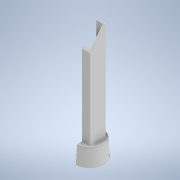
# Autodesk Inventor part: nozzle
Saved by Autodesk Inventor 2020.2 (Build 242310000, 310)
## iProperties
Created: 2020-09-23
Part Number: nozzle
Material: Generic
Document SubType Name: Modeling
Designer: Amaan Khalid
Density: 1 g/cm^3
Appearance: Default
Author: Amaan Khalid
Autodesk Inventor part; units mm, degrees
sketch "Sketch1" plane through (0, 0, 0) normal (1, 0, 0) x (0, 1, 0)
  line L0 (1.2879, 8.5778) -> (-61.8197, 8.5778)
  line L1 (-61.8197, 8.5778) -> (-61.8197, -4.1222)
  line L2 (-61.8197, -4.1222) -> (1.6803, -4.1222)
  line L3 (1.6803, -4.1222) -> (7.0029, -4.1222)
  line L4 (1.2879, 8.5778) -> (1.4492, 8.5778)
  line L5 (7.0029, -4.1222) -> (15.0709, -4.1222)
  line L6 (15.4791, -3.0007) -> (1.8574, 8.4293)
  arc A0 (1.8574, 8.4293) -> (1.4492, 8.5778) centre (1.4492, 7.9428) ccw
  arc A1 (15.0709, -4.1222) -> (15.4791, -3.0007) centre (15.0709, -3.4872) ccw
  point P0 (0, 0)
  point P1 (1.6803, 8.5778)
  point P2 (8.0303, -4.1222)
  dimension "d0" = 63.5
  dimension "d1" = 12.7
  dimension "d2" = 63.5
  dimension "d3" = 6.35
  dimension "d17" = 0.635
  constraints: 14 end point, 4 horizontal, 4 point on circle, 4 point on line, 4 tangent, 2 centre point, 1 equal radius, 1 perpendicular, 1 vertical
  measures "d0" distance of point (1.68, 8.578) L0.end
  measures "d1" distance of L0.end L1.end
  measures "d2" distance of L1.end L2.end
  measures "d3" distance of L2.end point (8.03, -4.122)
  measures "d17" radius of A0
extrude "Extrusion1" add sketch "Sketch1" along normal blind 12.7
sketch "Sketch2" plane through (0, -61.8197, -4.1222) normal (0, -1, 0) x (1, 0, 0)
  line L0 (12.7, 12.349) -> (12.7, 12.7) projected
  line L1 (0, 12.7) -> (0, 0) projected
  line L2 (12.7, 12.7) -> (0, 12.7)
  line L3 (0, 12.7) -> (0, 0)
  line L4 (0, 0) -> (12.7, 0)
  line L5 (12.7, 0) -> (12.7, 12.7)
  line L6 (11.43, 11.43) -> (1.27, 11.43)
  line L7 (1.27, 11.43) -> (1.27, 1.27)
  line L8 (1.27, 1.27) -> (11.43, 1.27)
  line L9 (11.43, 1.27) -> (11.43, 11.43)
  point P0 (0, 4.1222)
  dimension "d7" = 1.27
  constraints: 16 end point, 4 parallel, 2 perpendicular, 1 horizontal, 3 other
  measures "d7" distance between parallel lines of L5 L9
extrude "Extrusion2" cut sketch "Sketch2" against normal through all contours L9 L8 L7 L6
fillet "Fillet1" radius 0.635 14 edges at (12.7, -30.1852, 8.5778) (12.7, -61.8197, 2.2278) (12.7, -23.3744, -4.1222) (12.7, 15.6676, -3.7043) (12.7, 8.6682, 2.7143) (12.7, 1.6664, 8.5395) (0, -30.1852, 8.5778) (0, -61.8197, 2.2278) (0, -23.3744, -4.1222) (0, 15.6676, -3.7043) (0, 8.6682, 2.7143) (0, 1.6664, 8.5395) (6.35, -61.8197, 8.5778) (6.35, -61.8197, -4.1222)
ref_plane "Work Plane1" through (0, -63.5, 0) normal (0, 1, 0) x (-1, 0, 0)
sketch "Sketch6" plane through (0, -63.5, 0) normal (0, 1, 0) x (-1, 0, 0)
  circle A0 centre (-6.35, 2.2278) radius 10.0838
  line L0 (-11.43, 7.3078) -> (-1.27, 7.3078) projected
  line L1 (-1.27, 7.3078) -> (-11.43, 7.3078)
  line L2 (-11.43, -2.8522) -> (-11.43, 7.3078) projected
  line L3 (-11.43, 7.3078) -> (-11.43, -2.8522)
  line L4 (-11.43, -2.8522) -> (-1.27, -2.8522)
  line L5 (-1.27, 7.3078) -> (-1.27, -2.8522) projected
  line L6 (-1.27, -2.8522) -> (-1.27, 7.3078)
  point P0 (0, 0)
  point P1 (-1.905, 6.6728)
  point P2 (-1.905, -2.2172)
  point P3 (-10.795, 6.6728)
  point P4 (-10.795, -2.2172)
  point P5 (-1.27, -2.8522)
  constraints: 8 end point, 2 collinear, 1 centre point, 1 horizontal, 1 vertical
extrude "Extrusion4" add sketch "Sketch6" along normal up to surface (2.3153 mm away)
ref_plane "Work Plane2" through (0, 0, 2.2352) normal (0, 0, 1) x (1, 0, 0)
sketch "Sketch7" plane through (0, 0, 2.2352) normal (0, 0, 1) x (1, 0, 0)
  line L0 (-3.7338, -63.5) -> (-3.7338, -61.1847) projected
  line L1 (-3.7338, -63.5) -> (-3.7338, -71.12)
  line L2 (1.27, -63.5) -> (1.27, 3.1938) projected
  line L3 (-3.7338, -71.12) -> (1.27, -63.5)
  line L4 (0.635, -61.1847) -> (12.065, -61.1847) projected
  line L5 (6.35, -61.1847) -> (6.35, -66.8359)
  line L6 (-3.7338, -63.5) -> (1.27, -63.5)
  point P0 (0, 0)
  dimension "d21" = 7.62
  constraints: 8 end point, 1 collinear, 1 midpoint, 1 point on line, 1 vertical
  measures "d21" distance of L1.start L1.end
sketch "Sketch8" plane through (0, 0, 2.2352) normal (0, 0, 1) x (1, 0, 0)
  point P0 (0, 0)
sketch "Sketch9" plane through (0, 0, 2.2352) normal (0, 0, 1) x (1, 0, 0)
  point P0 (0, 0)
ref_plane "Work Plane3" through (0, 0, 0) normal (1, 0, 0) x (0, 1, 0)
sketch "Sketch10" plane through (0, 0, 0) normal (1, 0, 0) x (0, 1, 0)
  point P0 (0, 0)
ref_plane "Work Plane4" through (6.35, 0, 0) normal (1, 0, 0) x (0, 1, 0)
sketch "Sketch11" plane through (0, 0, 0) normal (1, 0, 0) x (0, 1, 0)
  point P0 (0, 0)
sketch "Sketch12" plane through (6.35, 0, 0) normal (1, 0, 0) x (0, 1, 0)
  line L0 (-63.5, 12.3116) -> (-61.1847, 12.3116) projected
  line L1 (-61.1847, 12.3116) -> (-73.5291, 12.3116)
  line L2 (-73.5291, 12.3116) -> (-73.5291, 13.226)
  line L3 (-63.5, -2.8522) -> (-63.5, 7.3078) projected
  line L4 (-63.5, 2.2278) -> (-67.3569, 2.2278)
  line L5 (-61.1847, 12.3116) -> (-61.1847, -7.856) projected
  line L6 (-61.1847, 12.3116) -> (-73.5291, 13.226)
  point P0 (0, 0)
  dimension "d27" = 12.3444
  dimension "d28" = 0.9144
  constraints: 8 end point, 2 horizontal, 1 midpoint, 1 vertical
  measures "d27" distance of L0.end L1.end
  measures "d28" distance of L1.end L2.end
revolve "Revolution2" add sketch "Sketch12" angle 360 about axis through (6.35, -63.5, 2.2278) along (0, -1, 0)
sketch "Sketch13" plane through (6.35, 0, 0) normal (1, 0, 0) x (0, 1, 0)
  line L0 (-63.5, 7.3078) -> (-63.5, -2.8522) projected
  line L1 (-63.5, 7.3078) -> (-67.0938, 12.3116)
  line L2 (-63.5, 12.3116) -> (-73.5291, 12.3116) projected
  line L3 (-63.5, 2.2278) -> (-65.2969, 2.2278)
  line L4 (-63.5, -7.856) -> (-63.5, 12.3116) projected
  line L5 (-63.5, 7.3078) -> (-63.5, 12.3116)
  line L6 (-63.5, 12.3116) -> (-67.0938, 12.3116)
  point P0 (0, 0)
  constraints: 8 end point, 2 collinear, 1 horizontal, 1 midpoint, 1 point on line
revolve "Revolution3" add sketch "Sketch13" angle 360 about axis through (6.35, -63.5, 2.2278) along (0, -1, 0)
ref_plane "Work Plane5" through (0, 60.325, 0) normal (0, 1, 0) x (-1, 0, 0)
sketch "Sketch14" plane through (0, 60.325, 0) normal (0, 1, 0) x (-1, 0, 0)
  line L0 (-11.43, -2.8522) -> (-11.43, 7.3078) projected
  line L1 (-11.43, -2.8522) -> (-11.43, 7.3078)
  line L2 (-11.43, 7.3078) -> (-1.27, 7.3078) projected
  line L3 (-11.43, 7.3078) -> (-1.27, 7.3078)
  line L4 (-1.27, 2.2278) -> (-1.27, -2.8522) projected
  line L5 (-1.27, 7.3078) -> (-1.27, -2.8522)
  line L6 (-1.27, -2.8522) -> (-11.43, -2.8522)
  point P0 (0, 0)
  constraints: 8 end point, 3 perpendicular, 1 vertical
extrude "Extrusion5" cut sketch "Sketch14" against normal blind 151.3166
sketch "Sketch15" plane through (6.35, 0, 0) normal (1, 0, 0) x (0, 1, 0)
  line L0 (-73.5291, -8.7704) -> (-73.5291, 13.226) projected
  line L1 (-73.5291, -8.7704) -> (-74.6755, -8.7704)
  line L2 (-74.6755, -8.7704) -> (-73.5291, -7.8583)
  line L3 (-73.5291, -8.7704) -> (-73.5291, -7.8583)
  line L4 (-73.5291, 2.2278) -> (-75.0963, 2.2278)
  point P0 (0, 0)
  constraints: 8 end point, 2 horizontal, 1 collinear, 1 midpoint, 1 point on line
revolve "Revolution4" add sketch "Sketch15" angle 360 about axis through (6.35, -73.5291, 2.2278) along (0, -1, 0)
equation "\"d2\" = d0"
body "Solid1"
